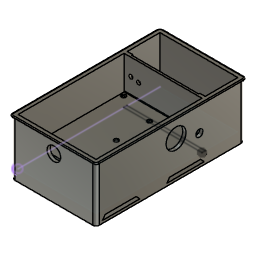
LED_BOX_bottom v31 (Autodesk Fusion 360 design; units mm, degrees)
Autodesk Fusion 360 part; units mm, degrees
sketch "Sketch1" plane through (0, 0, 0) normal (0, 0, 1) x (1, 0, 0)
  line L0 (0, 0) -> (65.4, 0)
  line L1 (65.4, 0) -> (65.4, 115)
  line L2 (65.4, 115) -> (0, 115)
  line L3 (0, 115) -> (0, 0)
  dimension "d1" = 115
  dimension "d7" = 65.4
  constraint horizontal L0
  constraint vertical L1
  constraint horizontal L2
  constraint vertical L3
  constraint coincident L0.start L3.end
  measures "d1" distance of L0.start L2.end
  measures "d7" distance of L0.start L0.end
extrude "Extrude1" add sketch "Sketch1" along normal blind 40 makes body 1
sketch "Sketch2" plane through (0, 0, 40) normal (0, 0, 1) x (-1, 0, 0)
  line L0 (0, -115) -> (0, 0)
  line L1 (0, 0) -> (-65.4, 0)
  line L2 (-65.4, 0) -> (-65.4, -115)
  line L3 (-65.4, -115) -> (0, -115)
  line L4 (-2.5, -112.5) -> (-62.9, -112.5)
  line L5 (-62.9, -112.5) -> (-62.9, -2.5)
  line L6 (-62.9, -2.5) -> (-2.5, -2.5)
  line L7 (-2.5, -2.5) -> (-2.5, -112.5)
  dimension "d4" = 110
  dimension "d5" = 60.4
  dimension "d6" = 2.5
  dimension "d8" = 2.5
  constraint horizontal L4
  constraint vertical L5
  constraint horizontal L6
  constraint vertical L7
  measures "d4" distance of L4.start L6.end
  measures "d5" distance of L5.end L6.end
  measures "d6" distance of L2.end L5
  measures "d8" distance of L3 L4
extrude "Extrude2" cut sketch "Sketch2" against normal blind 36.5 contours L4 L5 L6 L7 bodies 1
sketch "Sketch3" plane through (0, 0, 0) normal (0, -1, 0) x (1, 0, 0)
  line L0 (0, 0) -> (65.4, 0)
  line L1 (65.4, 0) -> (65.4, 40)
  line L2 (65.4, 40) -> (0, 40)
  line L3 (0, 40) -> (0, 0)
  circle A0 centre (32.7, 30) radius 5.3
  dimension "d11" = 10.6
  dimension "d12" = 32.7
  dimension "d13" = 30
  measures "d11" diameter of A0
  measures "d12" horizontal distance of L0.start A0.centre
  measures "d13" vertical distance of L0.start A0.centre
extrude "Extrude3" cut sketch "Sketch3" against normal blind 5 contours A0 bodies 1
sketch "Sketch4" plane through (0, 0, 3.5) normal (0, 0, 1) x (-1, 0, 0)
  line L0 (-2.5, -2.5) -> (-62.9, -2.5)
  line L1 (-62.9, -2.5) -> (-62.9, -112.5)
  line L2 (-62.9, -112.5) -> (-2.5, -112.5)
  line L3 (-2.2879, -87.2009) -> (-62.9, -87.2009)
  line L4 (-62.9, -87.2009) -> (-62.9, -84.7009)
  line L5 (-62.9, -84.7009) -> (-2.2879, -84.7009)
  line L6 (-2.2879, -84.7009) -> (-2.2879, -87.2009)
  line L7 (-2.5, -112.5) -> (-2.5, -2.5)
  dimension "d16" = 2.5
  dimension "d17" = 25.3
  constraint horizontal L3
  constraint vertical L4
  constraint horizontal L5
  constraint vertical L6
  constraint coincident L1 L4.end
  measures "d16" distance of L3.end L4.end
  measures "d17" distance of L2.end L3.start
extrude "Extrude4" add sketch "Sketch4" along normal blind 36.5 contours L1 L3 L4 L5 L7 | L3 L5 L6 L7 bodies 1
sketch "Sketch5" plane through (0, 0, 3.5) normal (0, 0, 1) x (-1, 0, 0)
  line L0 (-2.5, -87.2009) -> (-62.9, -87.2009)
  line L1 (-62.9, -87.2009) -> (-62.9, -112.5)
  line L2 (-62.9, -112.5) -> (-2.5, -112.5)
  line L3 (-7.7, -87.2009) -> (-57.7, -87.2009)
  line L4 (-57.7, -87.2009) -> (-57.7, -104.7009)
  line L5 (-57.7, -104.7009) -> (-7.7, -104.7009)
  line L6 (-7.7, -104.7009) -> (-7.7, -87.2009)
  circle A0 centre (-11.15, -101.2509) radius 4.5
  circle A1 centre (-54.25, -90.6509) radius 4.5
  line L7 (-2.5, -112.5) -> (-2.5, -87.2009)
  line L8 (-58.6, -86.3009) -> (-58.6, -105.6009)
  line L9 (-58.6, -105.6009) -> (-6.8, -105.6009)
  line L10 (-6.8, -105.6009) -> (-6.8, -86.3009)
  line L11 (-6.8, -86.3009) -> (-58.6, -86.3009)
  dimension "d20" = 50
  dimension "d21" = 17.5
  dimension "d24" = 3.45
  dimension "d25" = 3.45
  dimension "d27" = 3.45
  dimension "d28" = 3.45
  dimension "d29" = 9
  dimension "d30" = 9
  dimension "d63" = 5.2
  dimension "d177" = 0.9
  constraint horizontal L3
  constraint vertical L4
  constraint horizontal L5
  constraint vertical L6
  constraint coincident L0 L3.start
  measures "d20" distance of L3.start L3.end
  measures "d21" distance of L3.start L5.end
  measures "d24" distance of L4 A1.centre
  measures "d25" distance of L3 A1.centre
  measures "d27" distance of L6 A0.centre
  measures "d28" distance of L5 A0.centre
  measures "d29" diameter of A0
  measures "d30" diameter of A1
  measures "d63" horizontal distance of L2.end L5.end
extrude "Extrude5" add sketch "Sketch5" along normal blind 5 contours L6 A0 L10 | A0 L10 | L0 L3 L4 A1 | L0 L3 A1 L11 | L5 L6 A0 | A1 L11 | L5 A0 L9 | L4 A1 L8 | A0 L9 | A1 L8 picked at (-55.2541, -92.077) picked at (-9.9635, -102.2456) bodies 1
sketch "Sketch6" plane through (0, 0, 3.5) normal (0, 0, 1) x (-1, 0, 0)
  line L0 (-5.3, -111) -> (-15.8655, -88.3423)
  line L1 (-5.3, -111) -> (19.7, -111) construction
  line L2 (-15.8655, -88.3423) -> (-17.3655, -88.3423)
  line L3 (-17.3655, -88.3423) -> (-6.8, -111)
  line L4 (-6.8, -111) -> (-5.3, -111)
  line L5 (-2.5, -100.9) -> (-62.9, -100.9)
  line L6 (-62.9, -100.9) -> (-62.9, -98.9)
  line L7 (-62.9, -98.9) -> (-2.5, -98.9)
  line L8 (-2.5, -98.9) -> (-2.5, -100.9)
  line L9 (-62.9, -100.9) -> (-2.5, -100.9)
  point P0 (-2.5, -112.5)
  point P1 (-62.9, -112.5)
  dimension "d33" = 115
  dimension "d34" = 25
  dimension "d35" = 1.5
  dimension "d36" = 25
  dimension "d43" = 2
  dimension "d64" = 11.6
  dimension "d66" = 60.4
  constraint horizontal L1
  constraint horizontal L2
  constraint parallel L0 L3
  constraint horizontal L5
  constraint vertical L6
  constraint horizontal L7
  constraint vertical L8
  measures "d33" angle of L0 L1
  measures "d34" distance of L0.start L0.end
  measures "d35" distance of L0.end L2.end
  measures "d36" distance of L2.end L3.end
  measures "d43" distance of L5.start L7.end
  measures "d64" vertical distance of L5.start P0
  measures "d66" distance of L5.start L5.end
extrude "Extrude6" cut sketch "Sketch6" against normal blind 18 contours L0 L3 L4 L5 L9 | L0 L2 L3 L7 bodies 1
pattern_linear "R-Pattern1" count 11 spacing 4.4 along (1, 0, 0) of "Extrude6"
extrude "Extrude7" add sketch "Sketch5" along normal blind -3.5 and the other way blind -16.6 contours L6 A0 L10 | A0 L10 | L0 L3 L4 A1 | L0 L3 A1 L11 | L5 L6 A0 | A1 L11 | L5 A0 L9 | L4 A1 L8 | A0 L9 | A1 L8 picked at (-55.2541, -92.077) picked at (-9.9635, -102.2456) bodies 1
sketch "Sketch7" plane through (2.5, 0, 0) normal (1, 0, 0) x (0, 1, 0)
  line L0 (84.7009, 3.5) -> (84.7009, 40)
  line L1 (112.5, 40) -> (87.2009, 40)
  line L2 (87.2009, 40) -> (87.2009, 3.5)
  line L3 (87.2009, 3.5) -> (112.5, 3.5)
  line L4 (112.5, 3.5) -> (112.5, 40)
  line L5 (2.5, 40) -> (2.5, 3.5)
  line L6 (2.5, 3.5) -> (84.7009, 3.5)
  line L7 (84.7009, 14.05) -> (15.9009, 14.05)
  line L8 (15.9009, 14.05) -> (15.9009, 13.05)
  line L9 (15.9009, 13.05) -> (84.7009, 13.05)
  line L10 (84.7009, 13.05) -> (84.7009, 14.05)
  line L11 (15.9009, 14.05) -> (14.7009, 14.05)
  line L12 (14.7009, 14.05) -> (14.7009, 3.494)
  line L13 (14.7009, 3.494) -> (15.9009, 3.494)
  line L14 (15.9009, 3.494) -> (15.9009, 14.05)
  line L15 (84.7009, 40) -> (2.5, 40)
  dimension "d53" = 68.8
  dimension "d54" = 1
  dimension "d55" = 13.4009
  dimension "d56" = 9.55
  dimension "d57" = 1.2
  constraint horizontal L7
  constraint vertical L8
  constraint horizontal L9
  constraint vertical L10
  constraint coincident L0 L7.start
  constraint horizontal L11
  constraint vertical L12
  constraint horizontal L13
  constraint vertical L14
  measures "d53" distance of L7.start L7.end
  measures "d54" distance of L7.start L9.end
  measures "d55" distance of L5 L7.end
  measures "d56" distance of L6 L8.end
  measures "d57" distance of L7.end L11.end
extrude "Extrude8" add sketch "Sketch7" along normal blind 60.2 separate body contours L0 L7 L8 L9 L10 L14 | L6 L8 L11 L12 L14 makes body 2
sketch "Sketch8" plane through (0, 14.7009, 0) normal (0, -1, 0) x (1, 0, 0)
  line L0 (2.5, 14.05) -> (2.5, 3.5)
  line L1 (2.5, 3.5) -> (62.7, 3.5)
  line L2 (62.7, 3.5) -> (62.7, 14.05)
  line L3 (62.7, 14.05) -> (2.5, 14.05)
  circle A0 centre (9, 8) radius 3.125
  dimension "d60" = 6.25
  measures "d60" diameter of A0
extrude "Extrude9" cut sketch "Sketch8" against normal blind 3 contours A0 bodies 2
sketch "Sketch9" plane through (0, 0, 3.5) normal (0, 0, 1) x (-1, 0, 0)
  line L0 (-62.9, -84.7009) -> (-2.5, -84.7009)
  line L1 (-2.5, -84.7009) -> (-2.5, -2.5)
  line L2 (-2.5, -2.5) -> (-62.9, -2.5)
  line L3 (-62.9, -2.5) -> (-62.9, -84.7009)
  line L4 (-2.5, -14.5) -> (-3.5, -14.5)
  line L5 (-3.5, -14.5) -> (-3.5, -13.5)
  line L6 (-3.5, -13.5) -> (-2.5, -13.5)
  line L7 (-2.5, -13.5) -> (-2.5, -14.5)
  line L8 (-62.9, -13.5) -> (-61.9, -13.5)
  line L9 (-61.9, -13.5) -> (-61.9, -14.5)
  line L10 (-61.9, -14.5) -> (-62.9, -14.5)
  line L11 (-62.9, -14.5) -> (-62.9, -13.5)
  line L12 (-2.5, -83.2009) -> (-4, -83.2009)
  line L13 (-4, -83.2009) -> (-4, -84.7009)
  line L14 (-4, -84.7009) -> (-2.5, -84.7009)
  line L15 (-2.5, -84.7009) -> (-2.5, -83.2009)
  line L16 (-62.9, -84.7009) -> (-61.4, -84.7009)
  line L17 (-61.4, -84.7009) -> (-61.4, -83.2009)
  line L18 (-61.4, -83.2009) -> (-62.9, -83.2009)
  line L19 (-62.9, -83.2009) -> (-62.9, -84.7009)
  dimension "d67" = 1
  dimension "d68" = 1
  dimension "d69" = 60.4
  dimension "d70" = 12
  dimension "d71" = 12
  dimension "d94" = 1.5
  dimension "d95" = 1.5
  dimension "d96" = 1.5
  constraint horizontal L4
  constraint vertical L5
  constraint horizontal L6
  constraint vertical L7
  constraint coincident L1 L4.start
  constraint horizontal L8
  constraint vertical L9
  constraint horizontal L10
  constraint vertical L11
  constraint horizontal L12
  constraint vertical L13
  constraint horizontal L14
  constraint vertical L15
  constraint coincident L0.end L1.start
  constraint horizontal L18
  constraint vertical L19
  constraint horizontal L16
  constraint vertical L17
  measures "d67" distance of L4.start L4.end
  measures "d68" distance of L4.start L6.end
  measures "d69" horizontal distance of L4.start L10.end
  measures "d70" vertical distance of L2.end L9.end
  measures "d71" vertical distance of L1.end L4.end
  measures "d94" distance of L12.start L12.end
  measures "d95" distance of L0.end L12.start
  measures "d96" distance of L17.end L18.end
extrude "Extrude10" add sketch "Sketch9" along normal blind 9.55 contours L0 L3 L16 L17 L18 L19 | L0 L1 L12 L13 L14 L15 | L3 L8 L9 L10 L11 | L1 L4 L5 L6 L7 bodies 1
sketch "Sketch10" plane through (0, 0, 14.05) normal (0, 0, 1) x (-1, 0, 0)
  line L0 (-2.5, -14.7009) -> (-62.7, -14.7009)
  line L1 (-62.7, -14.7009) -> (-62.7, -84.7009)
  circle A0 centre (-5.1, -81.8009) radius 1.75
  circle A1 centre (-60.1, -81.8009) radius 1.75
  circle A2 centre (-58.4, -74.8759) radius 1.75
  circle A3 centre (-32, -74.8759) radius 1.75
  circle A4 centre (-58.4, -49.1759) radius 1.75
  circle A5 centre (-32, -49.1759) radius 1.75
  line L2 (-2.5, -84.7009) -> (-2.5, -14.7009)
  line L3 (-62.7, -84.7009) -> (-2.5, -84.7009)
  dimension "d74" = 3.5
  dimension "d77" = 3.5
  dimension "d78" = 2.6
  dimension "d80" = 3.5
  dimension "d81" = 4.3
  dimension "d83" = 3.5
  dimension "d84" = 30.7
  dimension "d86" = 3.5
  dimension "d87" = 4.3
  dimension "d89" = 3.5
  dimension "d91" = 30.7
  measures "d74" diameter of A0
  measures "d77" diameter of A1
  measures "d78" distance of L1 A1.centre
  measures "d80" diameter of A2
  measures "d81" distance of L1 A2.centre
  measures "d83" diameter of A3
  measures "d84" distance of L1 A3.centre
  measures "d86" diameter of A4
  measures "d87" distance of L1 A4.centre
  measures "d89" diameter of A5
  measures "d91" distance of L1 A5.centre
extrude "Extrude11" cut sketch "Sketch10" against normal blind 2 contours A0 | A1 | A2 | A3 | A4 | A5 bodies 2
sketch "Sketch11" plane through (2.5, 0, 0) normal (1, 0, 0) x (0, 1, 0)
  line L0 (14.5, 13.05) -> (14.5, 3.5)
  line L1 (84.7009, 13.05) -> (84.7009, 40)
  line L2 (84.7009, 40) -> (2.5, 40)
  line L3 (2.5, 40) -> (2.5, 3.5)
  line L4 (2.5, 3.5) -> (13.5, 3.5)
  line L5 (13.5, 3.5) -> (13.5, 13.05)
  line L6 (83.2009, 13.05) -> (84.7009, 13.05)
  line L7 (83.2009, 3.5) -> (83.2009, 13.05)
  line L8 (14.5, 3.5) -> (83.2009, 3.5)
  line L9 (13.5, 13.05) -> (14.5, 13.05)
sketch "Sketch12" plane through (2.5, 0, 0) normal (1, 0, 0) x (0, 1, 0)
  line L0 (84.7, 14.4) -> (84.45, 14.833)
  line L1 (84.7, 14.4) -> (85.2, 14.4) construction
  line L2 (84.45, 14.833) -> (84.7, 14.833)
  line L3 (84.7, 14.4) -> (84.7, 14.833)
  dimension "d97" = 120
  dimension "d98" = 0.5
  constraint horizontal L1
  constraint horizontal L2
  constraint perpendicular L2 L3
  measures "d97" angle of L0 L1
  measures "d98" distance of L0.start L0.end
extrude "Extrude12" add sketch "Sketch12" along normal blind 60.4 bodies 1
sketch "Sketch13" plane through (0, 84.7009, 0) normal (0, -1, 0) x (1, 0, 0)
  line L0 (2.5, 13.05) -> (4, 13.05)
  line L1 (4, 13.05) -> (4, 3.5)
  line L2 (4, 3.5) -> (61.4, 3.5)
  line L3 (61.4, 3.5) -> (61.4, 13.05)
  line L4 (61.4, 13.05) -> (62.9, 13.05)
  line L5 (62.9, 13.05) -> (62.9, 40)
  line L6 (62.9, 40) -> (2.5, 40)
  line L7 (2.5, 40) -> (2.5, 13.05)
  circle A0 centre (7.7, 26.833) radius 1.5
  line L8 (2.5, 40) -> (2.5, 3.5)
  circle A1 centre (57.7, 26.833) radius 1.75
  line L9 (2.5, 14.833) -> (62.9, 14.833)
  circle A2 centre (13.7, 25.833) radius 1.5
  dimension "d101" = 3
  dimension "d102" = 5.2
  dimension "d103" = 3.5
  dimension "d104" = 55.2
  dimension "d105" = 12
  dimension "d106" = 12
  dimension "d233" = 3
  dimension "d234" = 6
  dimension "d235" = 11
  measures "d101" diameter of A0
  measures "d102" distance of A0.centre L8
  measures "d103" diameter of A1
  measures "d104" distance of L8 A1.centre
  measures "d105" distance of A0.centre L9
  measures "d106" distance of A1.centre L9
  measures "d233" diameter of A2
  measures "d234" horizontal distance of A0.centre A2.centre
  measures "d235" distance of L9 A2.centre
extrude "Extrude13" cut sketch "Sketch13" against normal blind 5 contours A0 | A1 | A2 bodies 1
sketch "Sketch14" plane through (2.5, 0, 0) normal (1, 0, 0) x (0, 1, 0)
  line L0 (83.2009, 13.05) -> (84.7009, 13.05)
  line L1 (84.7009, 13.05) -> (84.7009, 40)
  line L2 (84.7009, 40) -> (2.5, 40)
  line L3 (2.5, 40) -> (2.5, 3.5)
  line L4 (2.5, 3.5) -> (13.5, 3.5)
  line L5 (13.5, 3.5) -> (13.5, 13.05)
  line L6 (13.5, 13.05) -> (14.5, 13.05)
  line L7 (14.5, 13.05) -> (14.5, 3.5)
  line L8 (14.5, 3.5) -> (83.2009, 3.5)
  line L9 (83.2009, 3.5) -> (83.2009, 13.05)
  circle A0 centre (17.5, 20.3) radius 2.5
  line L10 (84.7009, 14.05) -> (14.7009, 14.05)
  line L11 (84.45, 14.833) -> (84.7, 14.833)
  line L12 (84.7, 14.833) -> (84.7, 14.4)
  line L13 (84.7, 14.4) -> (84.45, 14.833)
  line L14 (2.5, 3.5) -> (17.5, 3.5)
  line L15 (17.5, 3.5) -> (17.5, 20.3)
  line L16 (17.5, 20.3) -> (2.5, 20.3)
  line L17 (2.5, 20.3) -> (2.5, 3.5)
  point P0 (14.7009, 14.05)
  dimension "d109" = 5
  dimension "d187" = 15
  dimension "d188" = 16.8
  constraint horizontal L14
  constraint vertical L15
  constraint horizontal L16
  constraint vertical L17
  constraint coincident A0.centre L15.end
  constraint coincident L3.end L4.start
  measures "d109" diameter of A0
  measures "d187" distance of A0.centre L16.end
  measures "d188" distance of L14.end A0.centre
extrude "Extrude14" cut sketch "Sketch14" against normal blind 10 contours A0 L15 L16 | A0 L15 L16 bodies 1
sketch "Sketch15" plane through (0, 0, 20.1) normal (0, 0, 1) x (-1, 0, 0)
  circle A0 centre (-54.25, -90.6509) radius 1.575
  circle A1 centre (-11.15, -101.2509) radius 1.575
  line L0 (-51.3608, -87.2009) -> (-57.1392, -87.2009)
  arc A2 (-57.1392, -87.2009) -> (-51.3608, -87.2009) centre (-54.25, -90.6509) ccw
  point P0 (-15.65, -101.2509)
  dimension "d120" = 3.15
  dimension "d123" = 3.15
  measures "d120" diameter of A0
  measures "d123" diameter of A1
sketch "Sketch16" plane through (0, 0, 40) normal (0, 0, 1) x (-1, 0, 0)
  line L0 (-62.9, -84.7009) -> (-62.9, -2.5)
  line L1 (-62.9, -2.5) -> (-2.5, -2.5)
  line L2 (-2.5, -2.5) -> (-2.5, -84.7009)
  line L3 (-2.5, -112.5) -> (-62.9, -112.5)
  line L4 (0, -115) -> (0, 0)
  line L5 (0, 0) -> (-65.4, 0)
  line L6 (-65.4, 0) -> (-65.4, -115)
  line L7 (-65.4, -115) -> (0, -115)
  line L8 (1, 1) -> (-66.4, 1)
  line L9 (-66.4, 1) -> (-66.4, -116)
  line L10 (-66.4, -116) -> (1, -116)
  line L11 (1, -116) -> (1, 1)
  line L12 (-2.5, -84.7009) -> (-62.9, -84.7009)
  line L13 (-62.9, -87.2009) -> (-2.5, -87.2009)
  line L14 (-2.5, -87.2009) -> (-2.5, -112.5)
  line L15 (-62.9, -112.5) -> (-62.9, -87.2009)
  dimension "d127" = 1
  dimension "d128" = 1
  dimension "d129" = 117
  dimension "d130" = 67.4
  constraint horizontal L8
  constraint vertical L9
  constraint horizontal L10
  constraint vertical L11
  measures "d127" horizontal distance of L4.end L8.start
  measures "d128" distance of L4.end L8
  measures "d129" distance of L8.start L10.end
  measures "d130" distance of L8.start L8.end
extrude "Extrude17" add sketch "Sketch16" against normal blind 1.5 contours L8 L9 L10 L11 bodies 1
fillet "Fillet2" radius 2.5 8 edges at (65.4, 0, 19.25) (0, 0, 19.25) (0, 115, 19.25) (65.4, 115, 19.25) (66.4, 116, 39.25) (66.4, -1, 39.25) (-1, -1, 39.25) (-1, 116, 39.25) on bodies 1
fillet "Fillet3" radius 1 16 edges at (65.6678, -0.2678, 38.5) (66.4, 57.5, 38.5) (65.6678, 115.2678, 38.5) (32.7, 116, 38.5) (-0.2678, 115.2678, 38.5) (-1, 57.5, 38.5) (-0.2678, -0.2678, 38.5) (32.7, -1, 38.5) (65.6678, 115.2678, 40) (66.4, 57.5, 40) (65.6678, -0.2678, 40) (32.7, -1, 40) (-0.2678, -0.2678, 40) (-1, 57.5, 40) (-0.2678, 115.2678, 40) (32.7, 116, 40) on bodies 1
extrude "Extrude19" cut sketch "Sketch5" along normal blind 38 contours L0 L3 A1 L10 L11 | L0 L3 A1 L11 | L0 L3 A1 L8 L11 bodies 1
sketch "Sketch19" plane through (62.9, 0, 0) normal (-1, 0, 0) x (0, -1, 0)
  line L0 (-13.5, 13.05) -> (-13.5, 3.5)
  line L1 (-13.5, 3.5) -> (-2.5, 3.5)
  line L2 (-2.5, 3.5) -> (-2.5, 40)
  line L3 (-2.5, 40) -> (-84.7009, 40)
  line L4 (-84.7009, 40) -> (-84.7009, 13.05)
  line L5 (-84.7009, 13.05) -> (-83.2009, 13.05)
  line L6 (-83.2009, 13.05) -> (-83.2009, 3.5)
  line L7 (-83.2009, 3.5) -> (-14.5, 3.5)
  line L8 (-14.5, 3.5) -> (-14.5, 13.05)
  line L9 (-14.5, 13.05) -> (-13.5, 13.05)
  circle A0 centre (-62.0759, 25.55) radius 7.75
  line L10 (-84.7009, 28.583) -> (-84.7009, 25.083)
  line L11 (-84.7009, 28.333) -> (-84.7009, 25.333)
  line L12 (-84.7009, 13.05) -> (-84.7009, 3.5)
  line L13 (-84.7009, 3.5) -> (-84.7009, 13.05)
  line L14 (-84.7009, 13.05) -> (-84.7009, 40)
  line L15 (-84.7009, 40) -> (-84.7009, 13.05)
  line L16 (-84.7009, 14.05) -> (-14.7009, 14.05)
  line L17 (-84.7, 14.833) -> (-84.45, 14.833)
  line L18 (-84.45, 14.833) -> (-84.7, 14.4)
  line L19 (-84.7, 14.4) -> (-84.7, 14.833)
  circle A1 centre (-80.2009, 20) radius 2.75
  line L20 (-84.7009, 27.333) -> (-84.7009, 24.333)
  dimension "d182" = 22.625
  dimension "d183" = 11.5
  dimension "d184" = 15.5
  dimension "d189" = 5.5
  dimension "d190" = 4.5
  measures "d182" distance of A0.centre L14
  measures "d183" distance of A0.centre L16
  measures "d184" diameter of A0
  measures "d189" diameter of A1
  measures "d190" distance of L14 A1.centre
extrude "Extrude20" cut sketch "Sketch19" against normal blind 2.5 contours A0 | A1 bodies 1
sketch "Sketch20" plane through (0, 0, 20.1) normal (0, 0, 1) x (-1, 0, 0)
  arc A0 (-57.1392, -87.2009) -> (-51.3608, -87.2009) centre (-54.25, -90.6509) ccw
  line L0 (-51.3608, -87.2009) -> (-57.1392, -87.2009)
  circle A1 centre (-11.15, -101.2509) radius 4.5
  line L1 (-12.7666, -98.4509) -> (-14.3832, -101.2509)
  line L2 (-14.3832, -101.2509) -> (-12.7666, -104.0509)
  line L3 (-12.7666, -104.0509) -> (-9.5334, -104.0509)
  line L4 (-9.5334, -104.0509) -> (-7.9168, -101.2509)
  line L5 (-7.9168, -101.2509) -> (-9.5334, -98.4509)
  line L6 (-9.5334, -98.4509) -> (-12.7666, -98.4509)
  line L7 (-52.6275, -93.4475) -> (-51.0168, -90.644)
  line L8 (-51.0168, -90.644) -> (-52.6394, -87.8475)
  line L9 (-52.6394, -87.8475) -> (-55.8725, -87.8543)
  line L10 (-55.8725, -87.8543) -> (-57.4832, -90.6577)
  line L11 (-57.4832, -90.6577) -> (-55.8606, -93.4543)
  line L12 (-55.8606, -93.4543) -> (-52.6275, -93.4475)
  circle A2 centre (-54.25, -90.6509) radius 2
  circle A3 centre (-11.15, -101.2509) radius 2
  point P0 (-11.15, -101.2509)
  point P1 (-11.15, -101.2509)
  point P2 (-54.25, -90.6509)
  point P3 (-54.25, -90.6509)
  dimension "d205" = 5.6
  dimension "d206" = 2.8
  dimension "d207" = 2.8
  dimension "d208" = 5.6
  dimension "d210" = 5.6
  dimension "d211" = 2.8
  dimension "d212" = 2.8
  dimension "d213" = 4
  dimension "d214" = 4
  constraint coincident P2 A0.centre
  constraint coincident P3 P2
  constraint concentric A1 A3
  measures "d205" distance of L2 L5
  measures "d206" distance of L5 P1
  measures "d207" distance of L1 P1
  measures "d208" vertical distance of L1.start L3.end
  measures "d210" distance of L9 L12
  measures "d211" distance of L7 P3
  measures "d212" distance of L9 P3
  measures "d213" diameter of A2
  measures "d214" diameter of A3
extrude "Extrude21" add sketch "Sketch5" along normal blind 16.6 contours L0 L3 A1 L11 | L4 A1 L8 bodies 1
extrude "Extrude22" cut sketch "Sketch20" against normal blind 2.8 contours L1 L2 L3 L4 L5 L6 | L7 L8 L9 L10 L11 L12 | A2 | A3 bodies 1
extrude "Extrude23" cut sketch "Sketch20" against normal blind 8 contours A2 | A3 bodies 1
extrude "Extrude24" add 1 faces at (32.9552, 31.1141, 0) along direction (0, 0, -1) blind 3 on bodies 1 bodies 1
sketch "Sketch21" plane through (0, 0, 0) normal (-1, 0, 0) x (0, -1, 0)
  circle A0 centre (-17.5, 20.3) radius 2.5
  line L0 (-112.5, 38.5) -> (-112.5, -3)
  line L1 (-112.5, -3) -> (-2.5, -3)
  line L2 (-2.5, -3) -> (-2.5, 38.5)
  line L3 (-2.5, 38.5) -> (-112.5, 38.5)
  line L4 (-5, -1) -> (-34, -1)
  line L5 (-5, -1) -> (-7.1006, 2)
  line L6 (-5, -1) -> (-1.3377, -1) construction
  line L7 (-34, -1) -> (-31, 2)
  line L8 (-34, -1) -> (-31, -1) construction
  line L9 (-31, 2) -> (-7.1006, 2)
  dimension "d219" = 2
  dimension "d221" = 125
  dimension "d222" = 3
  dimension "d223" = 45
  dimension "d225" = 3
  dimension "d228" = 2.5
  constraint horizontal L4
  constraint horizontal L6
  constraint horizontal L8
  constraint horizontal L9
  measures "d219" distance of L1 L4
  measures "d221" angle of L5 L6
  measures "d222" vertical distance of L4.start L5.end
  measures "d223" angle of L7 L8
  measures "d225" distance of L4 L7.end
  measures "d228" distance of L2 L4.start
extrude "Extrude25" cut sketch "Sketch21" against normal blind 89 contours L4 L5 L7 L9 bodies 1
pattern_linear "R-Pattern3" count 2 spacing 50 along (0, 1, 0) of "Extrude25"
equation "d183 = 4 mm + 7.5 mm"
named bodies: "Box_bottom", "Cover_lithium_battery"
